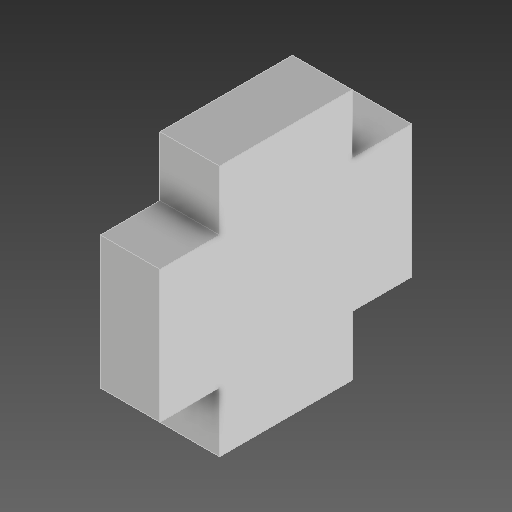
# Autodesk Inventor part: Inner Rib
Saved by Autodesk Inventor 2020.1 (Build 241239000, 239)
## iProperties
Created: 2019-08-27
Part Number: Inner Rib
Material: Generic
Document SubType Name: Modeling
Designer: Oliver Frolovs
Density: 1 g/cm^3
Appearance: Default
Mass: 10.08 g
Surface Area: 36.08 cm^2
Volume: 10.08 cm^3
Author: Oliver Frolovs
Autodesk Inventor part; units mm, degrees
ref_plane "YZ Plane" through (0, 0, 0) normal (1, 0, 0) x (0, 1, 0)
ref_plane "XZ Plane" through (0, 0, 0) normal (0, 1, 0) x (-1, 0, 0)
ref_plane "XY Plane" through (0, 0, 0) normal (0, 0, 1) x (1, 0, 0)
sketch "Inner Rib Profile" plane through (0, 0, 0) normal (1, 0, 0) x (0, 1, 0)
  line L0 (-10, 10) -> (10, 10) construction
  line L1 (10, 10) -> (10, -10) construction
  line L2 (10, -10) -> (-10, -10) construction
  line L3 (-10, -10) -> (-10, 10) construction
  line L4 (-10, 10) -> (10, -10) construction
  line L5 (10, 10) -> (-10, -10) construction
  line L6 (-10, -10) -> (-10, -19)
  line L7 (-10, -19) -> (10, -19)
  line L8 (10, -19) -> (10, -10)
  line L9 (0, 0) -> (-10, 0) construction
  line L10 (-10, 10) -> (-10, 19)
  line L11 (-10, 19) -> (10, 19)
  line L12 (10, 19) -> (10, 10)
  line L13 (-10, 10) -> (-19, 10)
  line L14 (-19, 10) -> (-19, -10)
  line L15 (-19, -10) -> (-10, -10)
  line L16 (0, 0) -> (0, 10) construction
  line L17 (10, 10) -> (19, 10)
  line L18 (19, 10) -> (19, -10)
  line L19 (19, -10) -> (10, -10)
  dimension "d0" = 20
  dimension "d1" = 20
  dimension "d2" = 9
  dimension "d3" = 9
  constraints: 40 end point, 6 perpendicular, 5 midpoint, 4 symmetric about line, 3 horizontal, 1 coincident, 1 parallel
  measures "d0" distance of L0.end L1.end
  measures "d1" distance of L1.end L2.end
  measures "d2" distance of L7.end L1.end
  measures "d3" distance of L14.end L2.end
extrude "Make Inner Rib by Extrusion of Its Profile" add sketch "Inner Rib Profile" along normal mid plane 9
sketch "Laser Cutter Sketch" plane through (4.5, 0, 0) normal (1, 0, 0) x (0, 0, -1)
  line L0 (-19, 10) -> (-19, -10) construction
  line L1 (-19, -10) -> (-10, -10) construction
  line L2 (-10, -10) -> (-10, -19) projected
  line L3 (-10, -19) -> (10, -19) projected
  line L4 (10, -19) -> (10, -10) projected
  line L5 (10, -10) -> (19, -10) construction
  line L6 (19, -10) -> (19, 10) construction
  line L7 (19, 10) -> (10, 10) construction
  line L8 (10, 10) -> (10, 19) projected
  line L9 (10, 19) -> (-10, 19) projected
  line L10 (-10, 19) -> (-10, 10) projected
  line L11 (-10, 10) -> (-19, 10) construction
  line L12 (0, 0) -> (0, 19) construction
  line L13 (-5, 0) -> (5, 0) construction
  line L14 (-5, -2.5) -> (5, -2.5)
  line L15 (5, 2.5) -> (-5, 2.5)
  arc A0 (-5, 2.5) -> (-5, -2.5) centre (-5, 0) ccw
  arc A1 (5, -2.5) -> (5, 2.5) centre (5, 0) ccw
  line L16 (10, -10.25) -> (19.25, -10.25)
  line L17 (19.25, -10.25) -> (19.25, 10.25)
  line L18 (19.25, 10.25) -> (10, 10.25)
  line L19 (-10, -10.25) -> (-19.25, -10.25)
  line L20 (-19.25, -10.25) -> (-19.25, 10.25)
  line L21 (-19.25, 10.25) -> (-10, 10.25)
  line L22 (-10, -19) -> (-10, -10.25)
  line L23 (-10, 19) -> (-10, 10.25)
  line L24 (10, -10.25) -> (10, -19)
  line L25 (10, 10.25) -> (10, 19)
  dimension "d7" = 10
  dimension "d8" = 5
  dimension "d13" = 0.25
  constraints: 30 end point, 4 point on circle, 4 symmetric about line, 4 tangent, 3 point on line, 2 centre point, 2 midpoint, 1 coincident, 1 parallel, 1 perpendicular, 2 other
  measures "d7" distance of L15.start L15.end
  measures "d8" distance between parallel lines of L14 L15
  measures "d13" distance between parallel lines of L5 L16
equation "\"d0\" = InnerRibHeight"
equation "\"d1\" = RibSlotLength"
equation "\"d2\" = PrototypePlateMaterialThickness"
equation "\"d4\" = PrototypePlateRibMaterialThickness"
equation "\"InnerRibHeight\" = 20"
equation "\"RibSlotLength\" = 20"
equation "\"PrototypePlateMaterialThickness\" = 9"
equation "\"PrototypePlateRibMaterialThickness\" = 9"
body "Solid1"
